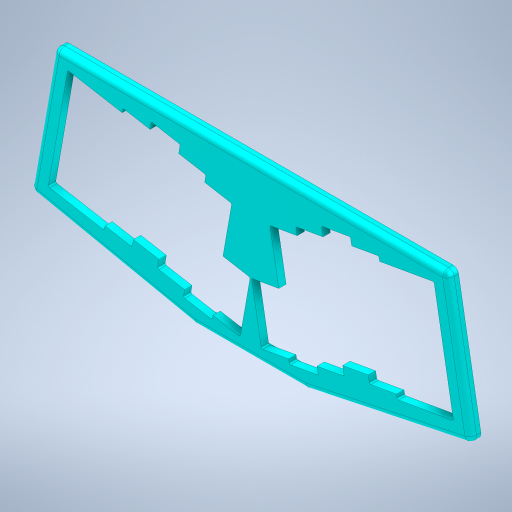
# Autodesk Inventor part: top-case
Saved by Autodesk Inventor 2023 (Build 270158000, 158)
## iProperties
Created: 2022-09-10
Part Number: top-case
Material: Aluminum 6061-AHC
Document SubType Name: Modeling
Designer: hainguyen
Density: 2.7 g/cm^3
Appearance: Aluminum - Dark
Author: hainguyen
Autodesk Inventor part; units mm, degrees
(part 1 of 2)
ref_plane "YZ Plane" through (0, 0, 0) normal (1, 0, 0) x (0, 1, 0)
ref_plane "XZ Plane" through (0, 0, 0) normal (0, 1, 0) x (-1, 0, 0)
ref_plane "XY Plane" through (0, 0, 0) normal (0, 0, 1) x (1, 0, 0)
sketch "Sketch1" plane through (0, 0, 0) normal (0, 0, 1) x (1, 0, 0)
  line L0 (125.9391, 53.8097) -> (-64.6396, 53.8097) construction
  line L1 (191.9239, 53.9833) -> (205.6869, -24.0807) construction
  line L2 (164.2137, -32.7433) -> (204.7021, -24.2544) construction
  line L3 (-64.6396, 53.8097) -> (-78.4038, -24.2539) construction
  line L4 (-78.4038, -24.2539) -> (-37.9155, -32.743) construction
  line L5 (25.7012, -46.0813) -> (100.5969, -46.0813) construction
  line L6 (-72.1915, 62.8097) -> (198.4911, 62.8097)
  line L7 (198.4911, 62.8097) -> (215.0786, -31.2745)
  line L8 (215.0786, -31.2745) -> (101.5302, -55.0813)
  line L9 (101.5302, -55.0813) -> (24.7678, -55.0813)
  line L10 (24.7678, -55.0813) -> (-88.7804, -31.274)
  line L11 (-88.7804, -31.274) -> (-72.1915, 62.8097)
  line L12 (204.7021, -24.2544) -> (190.9391, 53.8097) construction
  point P0 (0, 0)
extrude "Extrusion1" add sketch "Sketch1" along normal blind 7
sketch "Sketch2" plane through (0, 0, 0) normal (0, 0, -1) x (-1, 0, 0)
  arc A0 (47.2919, 31.2612) -> (47.5236, 31.0989) centre (47.4889, 31.2959) ccw construction
  line L0 (65.0532, 34.1898) -> (47.5236, 31.0989) construction
  arc A1 (65.0532, 34.1898) -> (65.2154, 34.4214) centre (65.0185, 34.3867) ccw construction
  line L1 (62.1246, 51.951) -> (65.2154, 34.4214) construction
  arc A2 (62.1246, 51.951) -> (61.8929, 52.1133) centre (61.9276, 51.9163) ccw construction
  line L2 (44.3633, 49.0224) -> (61.8929, 52.1133) construction
  arc A3 (44.3633, 49.0224) -> (44.2011, 48.7907) centre (44.398, 48.8255) ccw construction
  line L3 (47.2919, 31.2612) -> (44.2011, 48.7907) construction
  line L4 (63.1649, 35.6846) -> (48.7867, 33.1494) construction
  line L5 (48.7867, 33.1494) -> (46.2516, 47.5276) construction
  line L6 (46.2516, 47.5276) -> (60.6298, 50.0628) construction
  line L7 (60.6298, 50.0628) -> (63.1649, 35.6846) construction
  arc A4 (28.5806, 27.9618) -> (28.8122, 27.7996) centre (28.7775, 27.9966) ccw construction
  line L8 (46.3418, 30.8904) -> (28.8122, 27.7996) construction
  arc A5 (46.3418, 30.8904) -> (46.5041, 31.1221) centre (46.3071, 31.0874) ccw construction
  line L9 (43.4132, 48.6517) -> (46.5041, 31.1221) construction
  arc A6 (43.4132, 48.6517) -> (43.1816, 48.814) centre (43.2163, 48.617) ccw construction
  line L10 (25.652, 45.7231) -> (43.1816, 48.814) construction
  arc A7 (25.652, 45.7231) -> (25.4897, 45.4914) centre (25.6867, 45.5262) ccw construction
  line L11 (28.5806, 27.9618) -> (25.4897, 45.4914) construction
  line L12 (44.4536, 32.3853) -> (30.0754, 29.8501) construction
  line L13 (30.0754, 29.8501) -> (27.5402, 44.2283) construction
  line L14 (27.5402, 44.2283) -> (41.9184, 46.7635) construction
  line L15 (41.9184, 46.7635) -> (44.4536, 32.3853) construction
  arc A8 (9.3483, 27.6169) -> (9.58, 27.4547) centre (9.5452, 27.6517) ccw construction
  line L16 (27.1096, 30.5455) -> (9.58, 27.4547) construction
  arc A9 (27.1096, 30.5455) -> (27.2718, 30.7772) centre (27.0748, 30.7425) ccw construction
  line L17 (24.1809, 48.3068) -> (27.2718, 30.7772) construction
  arc A10 (24.1809, 48.3068) -> (23.9493, 48.4691) centre (23.984, 48.2721) ccw construction
  line L18 (6.4197, 45.3782) -> (23.9493, 48.4691) construction
  arc A11 (6.4197, 45.3782) -> (6.2574, 45.1465) centre (6.4544, 45.1813) ccw construction
  line L19 (9.3483, 27.6169) -> (6.2574, 45.1465) construction
  line L20 (25.2213, 32.0404) -> (10.8431, 29.5052) construction
  line L21 (10.8431, 29.5052) -> (8.3079, 43.8834) construction
  line L22 (8.3079, 43.8834) -> (22.6861, 46.4186) construction
  line L23 (22.6861, 46.4186) -> (25.2213, 32.0404) construction
  arc A12 (-10.2313, 29.2417) -> (-9.9996, 29.0794) centre (-10.0344, 29.2764) ccw construction
  line L24 (7.53, 32.1703) -> (-9.9996, 29.0794) construction
  arc A13 (7.53, 32.1703) -> (7.6922, 32.402) centre (7.4952, 32.3672) ccw construction
  line L25 (4.6014, 49.9316) -> (7.6922, 32.402) construction
  arc A14 (4.6014, 49.9316) -> (4.3697, 50.0938) centre (4.4044, 49.8968) ccw construction
  line L26 (-13.1599, 47.003) -> (4.3697, 50.0938) construction
  arc A15 (-13.1599, 47.003) -> (-13.3222, 46.7713) centre (-13.1252, 46.806) ccw construction
  line L27 (-10.2313, 29.2417) -> (-13.3222, 46.7713) construction
  line L28 (5.6417, 33.6651) -> (-8.7365, 31.1299) construction
  line L29 (-8.7365, 31.1299) -> (-11.2717, 45.5081) construction
  line L30 (-11.2717, 45.5081) -> (3.1065, 48.0433) construction
  line L31 (3.1065, 48.0433) -> (5.6417, 33.6651) construction
  arc A16 (-27.9008, 20.0335) -> (-27.6691, 19.8713) centre (-27.7038, 20.0682) ccw construction
  line L32 (-10.1395, 22.9621) -> (-27.6691, 19.8713) construction
  arc A17 (-10.1395, 22.9621) -> (-9.9773, 23.1938) centre (-10.1742, 23.1591) ccw construction
  line L33 (-13.0681, 40.7234) -> (-9.9773, 23.1938) construction
  arc A18 (-13.0681, 40.7234) -> (-13.2998, 40.8856) centre (-13.2651, 40.6887) ccw construction
  line L34 (-30.8294, 37.7948) -> (-13.2998, 40.8856) construction
  arc A19 (-30.8294, 37.7948) -> (-30.9916, 37.5631) centre (-30.7947, 37.5978) ccw construction
  line L35 (-27.9008, 20.0335) -> (-30.9916, 37.5631) construction
  line L36 (-12.0277, 24.4569) -> (-26.406, 21.9218) construction
  line L37 (-26.406, 21.9218) -> (-28.9411, 36.3) construction
  line L38 (-28.9411, 36.3) -> (-14.5629, 38.8351) construction
  line L39 (-14.5629, 38.8351) -> (-12.0277, 24.4569) construction
  arc A20 (-45.7439, 11.8102) -> (-45.5122, 11.6479) centre (-45.5469, 11.8449) ccw construction
  line L40 (-27.9826, 14.7388) -> (-45.5122, 11.6479) construction
  arc A21 (-27.9826, 14.7388) -> (-27.8204, 14.9704) centre (-28.0173, 14.9357) ccw construction
  line L41 (-30.9112, 32.5) -> (-27.8204, 14.9704) construction
  arc A22 (-30.9112, 32.5) -> (-31.1429, 32.6623) centre (-31.1082, 32.4653) ccw construction
  line L42 (-48.6725, 29.5714) -> (-31.1429, 32.6623) construction
  arc A23 (-48.6725, 29.5714) -> (-48.8347, 29.3397) centre (-48.6378, 29.3745) ccw construction
  line L43 (-45.7439, 11.8102) -> (-48.8347, 29.3397) construction
  line L44 (-29.8709, 16.2336) -> (-44.2491, 13.6984) construction
  line L45 (-44.2491, 13.6984) -> (-46.7842, 28.0766) construction
  line L46 (-46.7842, 28.0766) -> (-32.406, 30.6118) construction
  line L47 (-32.406, 30.6118) -> (-29.8709, 16.2336) construction
  arc A24 (-55.0778, -44.6518) -> (-54.8461, -44.8141) centre (-54.8809, -44.6171) ccw construction
  line L48 (-37.3165, -41.7232) -> (-54.8461, -44.8141) construction
  arc A25 (-37.3165, -41.7232) -> (-37.1543, -41.4916) centre (-37.3513, -41.5263) ccw construction
  line L49 (-40.2451, -23.962) -> (-37.1543, -41.4916) construction
  arc A26 (-40.2451, -23.962) -> (-40.4768, -23.7997) centre (-40.4421, -23.9967) ccw construction
  line L50 (-58.0064, -26.8906) -> (-40.4768, -23.7997) construction
  arc A27 (-58.0064, -26.8906) -> (-58.1687, -27.1222) centre (-57.9717, -27.0875) ccw construction
  line L51 (-55.0778, -44.6518) -> (-58.1687, -27.1222) construction
  line L52 (-39.2048, -40.2284) -> (-53.583, -42.7636) construction
  line L53 (-53.583, -42.7636) -> (-56.1182, -28.3854) construction
  line L54 (-56.1182, -28.3854) -> (-41.74, -25.8502) construction
  line L55 (-41.74, -25.8502) -> (-39.2048, -40.2284) construction
  arc A28 (-58.3751, -25.9518) -> (-58.1435, -26.1141) centre (-58.1782, -25.9171) ccw construction
  line L56 (-40.6139, -23.0232) -> (-58.1435, -26.1141) construction
  arc A29 (-40.6139, -23.0232) -> (-40.4516, -22.7916) centre (-40.6486, -22.8263) ccw construction
  line L57 (-43.5425, -5.262) -> (-40.4516, -22.7916) construction
  arc A30 (-43.5425, -5.262) -> (-43.7741, -5.0997) centre (-43.7394, -5.2967) ccw construction
  line L58 (-61.3037, -8.1906) -> (-43.7741, -5.0997) construction
  arc A31 (-61.3037, -8.1906) -> (-61.466, -8.4222) centre (-61.269, -8.3875) ccw construction
  line L59 (-58.3751, -25.9518) -> (-61.466, -8.4222) construction
  line L60 (-42.5021, -21.5284) -> (-56.8803, -24.0636) construction
  line L61 (-56.8803, -24.0636) -> (-59.4155, -9.6854) construction
  line L62 (-59.4155, -9.6854) -> (-45.0373, -7.1502) construction
  line L63 (-45.0373, -7.1502) -> (-42.5021, -21.5284) construction
  arc A32 (-35.8459, -44.3239) -> (-35.6143, -44.4861) centre (-35.649, -44.2892) ccw construction
  line L64 (-18.0847, -41.3953) -> (-35.6143, -44.4861) construction
  arc A33 (-18.0847, -41.3953) -> (-17.9224, -41.1636) centre (-18.1194, -41.1983) ccw construction
  line L65 (-21.0133, -23.634) -> (-17.9224, -41.1636) construction
  arc A34 (-21.0133, -23.634) -> (-21.2449, -23.4718) centre (-21.2102, -23.6687) ccw construction
  line L66 (-38.7745, -26.5626) -> (-21.2449, -23.4718) construction
  arc A35 (-38.7745, -26.5626) -> (-38.9368, -26.7943) centre (-38.7398, -26.7596) ccw construction
  line L67 (-35.8459, -44.3239) -> (-38.9368, -26.7943) construction
  line L68 (-19.9729, -39.9005) -> (-34.3511, -42.4356) construction
  line L69 (-34.3511, -42.4356) -> (-36.8863, -28.0574) construction
  line L70 (-36.8863, -28.0574) -> (-22.5081, -25.5223) construction
  line L71 (-22.5081, -25.5223) -> (-19.9729, -39.9005) construction
  arc A36 (-18.0028, -36.1005) -> (-17.7711, -36.2628) centre (-17.8059, -36.0658) ccw construction
  line L72 (-0.2415, -33.1719) -> (-17.7711, -36.2628) construction
  arc A37 (-0.2415, -33.1719) -> (-0.0793, -32.9402) centre (-0.2763, -32.975) ccw construction
  line L73 (-3.1702, -15.4106) -> (-0.0793, -32.9402) construction
  arc A38 (-3.1702, -15.4106) -> (-3.4018, -15.2484) centre (-3.3671, -15.4454) ccw construction
  line L74 (-20.9314, -18.3392) -> (-3.4018, -15.2484) construction
  arc A39 (-20.9314, -18.3392) -> (-21.0937, -18.5709) centre (-20.8967, -18.5362) ccw construction
  line L75 (-18.0028, -36.1005) -> (-21.0937, -18.5709) construction
  line L76 (-2.1298, -31.6771) -> (-16.508, -34.2123) construction
  line L77 (-16.508, -34.2123) -> (-19.0432, -19.8341) construction
  line L78 (-19.0432, -19.8341) -> (-4.665, -17.2989) construction
  line L79 (-4.665, -17.2989) -> (-2.1298, -31.6771) construction
  arc A40 (-0.3334, -26.8924) -> (-0.1017, -27.0546) centre (-0.1364, -26.8576) ccw construction
  line L80 (17.4279, -23.9638) -> (-0.1017, -27.0546) construction
  arc A41 (17.4279, -23.9638) -> (17.5901, -23.7321) centre (17.3932, -23.7668) ccw construction
  line L81 (14.4993, -6.2025) -> (17.5901, -23.7321) construction
  arc A42 (14.4993, -6.2025) -> (14.2676, -6.0403) centre (14.3023, -6.2372) ccw construction
  line L82 (-3.262, -9.1311) -> (14.2676, -6.0403) construction
  arc A43 (-3.262, -9.1311) -> (-3.4242, -9.3628) centre (-3.2273, -9.328) ccw construction
  line L83 (-0.3334, -26.8924) -> (-3.4242, -9.3628) construction
  line L84 (15.5397, -22.4689) -> (1.1615, -25.0041) construction
  line L85 (1.1615, -25.0041) -> (-1.3737, -10.6259) construction
  line L86 (-1.3737, -10.6259) -> (13.0045, -8.0907) construction
  line L87 (13.0045, -8.0907) -> (15.5397, -22.4689) construction
  arc A44 (19.2462, -28.5171) -> (19.4779, -28.6793) centre (19.4432, -28.4824) ccw construction
  line L88 (37.0075, -25.5885) -> (19.4779, -28.6793) construction
  arc A45 (37.0075, -25.5885) -> (37.1697, -25.3568) centre (36.9728, -25.3915) ccw construction
  line L89 (34.0789, -7.8272) -> (37.1697, -25.3568) construction
  arc A46 (34.0789, -7.8272) -> (33.8472, -7.665) centre (33.8819, -7.8619) ccw construction
  line L90 (16.3176, -10.7558) -> (33.8472, -7.665) construction
  arc A47 (16.3176, -10.7558) -> (16.1554, -10.9875) centre (16.3523, -10.9528) ccw construction
  line L91 (19.2462, -28.5171) -> (16.1554, -10.9875) construction
  line L92 (35.1192, -24.0937) -> (20.741, -26.6288) construction
  line L93 (20.741, -26.6288) -> (18.2059, -12.2506) construction
  line L94 (18.2059, -12.2506) -> (32.5841, -9.7155) construction
  line L95 (32.5841, -9.7155) -> (35.1192, -24.0937) construction
  arc A48 (38.4785, -28.1722) -> (38.7102, -28.3344) centre (38.6755, -28.1375) ccw construction
  line L96 (56.2398, -25.2436) -> (38.7102, -28.3344) construction
  arc A49 (56.2398, -25.2436) -> (56.402, -25.0119) centre (56.2051, -25.0466) ccw construction
  line L97 (53.3112, -7.4823) -> (56.402, -25.0119) construction
  arc A50 (53.3112, -7.4823) -> (53.0795, -7.3201) centre (53.1142, -7.517) ccw construction
  line L98 (35.5499, -10.4109) -> (53.0795, -7.3201) construction
  arc A51 (35.5499, -10.4109) -> (35.3877, -10.6426) centre (35.5846, -10.6079) ccw construction
  line L99 (38.4785, -28.1722) -> (35.3877, -10.6426) construction
  line L100 (54.3515, -23.7488) -> (39.9733, -26.284) construction
  line L101 (39.9733, -26.284) -> (37.4382, -11.9057) construction
  line L102 (37.4382, -11.9057) -> (51.8164, -9.3706) construction
  line L103 (51.8164, -9.3706) -> (54.3515, -23.7488) construction
  arc A52 (57.1899, -24.8729) -> (57.4215, -25.0351) centre (57.3868, -24.8382) ccw construction
  line L104 (74.9511, -21.9443) -> (57.4215, -25.0351) construction
  arc A53 (74.9511, -21.9443) -> (75.1134, -21.7126) centre (74.9164, -21.7473) ccw construction
  line L105 (72.0225, -4.183) -> (75.1134, -21.7126) construction
  arc A54 (72.0225, -4.183) -> (71.7908, -4.0208) centre (71.8256, -4.2177) ccw construction
  line L106 (54.2612, -7.1116) -> (71.7908, -4.0208) construction
  arc A55 (54.2612, -7.1116) -> (54.099, -7.3433) centre (54.296, -7.3086) ccw construction
  line L107 (57.1899, -24.8729) -> (54.099, -7.3433) construction
  line L108 (73.0629, -20.4495) -> (58.6847, -22.9846) construction
  line L109 (58.6847, -22.9846) -> (56.1495, -8.6064) construction
  line L110 (56.1495, -8.6064) -> (70.5277, -6.0713) construction
  line L111 (70.5277, -6.0713) -> (73.0629, -20.4495) construction
  arc A56 (-88.9737, -41.5091) -> (-88.8115, -41.7408) centre (-88.7767, -41.5438) ccw construction
  line L112 (-71.2818, -44.8313) -> (-88.8115, -41.7408) construction
  arc A57 (-71.2818, -44.8313) -> (-71.0501, -44.6691) centre (-71.2471, -44.6344) ccw construction
  line L113 (-67.9596, -27.1394) -> (-71.0501, -44.6691) construction
  arc A58 (-67.9596, -27.1394) -> (-68.1218, -26.9078) centre (-68.1565, -27.1047) ccw construction
  line L114 (-85.6515, -23.8172) -> (-68.1218, -26.9078) construction
  arc A59 (-85.6515, -23.8172) -> (-85.8832, -23.9794) centre (-85.6862, -24.0142) ccw construction
  line L115 (-88.9737, -41.5091) -> (-85.8832, -23.9794) construction
  line L116 (-72.545, -42.7809) -> (-86.9232, -40.2459) construction
  line L117 (-86.9232, -40.2459) -> (-84.3883, -25.8677) construction
  line L118 (-84.3883, -25.8677) -> (-70.01, -28.4026) construction
  line L119 (-70.01, -28.4026) -> (-72.545, -42.7809) construction
  arc A60 (-108.2002, -41.175) -> (-108.038, -41.4067) centre (-108.0033, -41.2098) ccw construction
  line L120 (-90.5084, -44.4973) -> (-108.038, -41.4067) construction
  arc A61 (-90.5084, -44.4973) -> (-90.2767, -44.335) centre (-90.4736, -44.3003) ccw construction
  line L121 (-87.1861, -26.8054) -> (-90.2767, -44.335) construction
  arc A62 (-87.1861, -26.8054) -> (-87.3484, -26.5737) centre (-87.3831, -26.7707) ccw construction
  line L122 (-104.878, -23.4831) -> (-87.3484, -26.5737) construction
  arc A63 (-104.878, -23.4831) -> (-105.1097, -23.6454) centre (-104.9127, -23.6801) ccw construction
  line L123 (-108.2002, -41.175) -> (-105.1097, -23.6454) construction
  line L124 (-91.7715, -42.4468) -> (-106.1498, -39.9119) construction
  line L125 (-106.1498, -39.9119) -> (-103.6148, -25.5336) construction
  line L126 (-103.6148, -25.5336) -> (-89.2366, -28.0686) construction
  line L127 (-89.2366, -28.0686) -> (-91.7715, -42.4468) construction
  arc A64 (-126.0433, -32.9517) -> (-125.8811, -33.1834) centre (-125.8464, -32.9864) ccw construction
  line L128 (-108.3515, -36.2739) -> (-125.8811, -33.1834) construction
  arc A65 (-108.3515, -36.2739) -> (-108.1198, -36.1117) centre (-108.3167, -36.077) ccw construction
  line L129 (-105.0292, -18.582) -> (-108.1198, -36.1117) construction
  arc A66 (-105.0292, -18.582) -> (-105.1915, -18.3503) centre (-105.2262, -18.5473) ccw construction
  line L130 (-122.7211, -15.2598) -> (-105.1915, -18.3503) construction
  arc A67 (-122.7211, -15.2598) -> (-122.9528, -15.422) centre (-122.7558, -15.4568) ccw construction
  line L131 (-126.0433, -32.9517) -> (-122.9528, -15.422) construction
  line L132 (-109.6146, -34.2235) -> (-123.9929, -31.6885) construction
  line L133 (-123.9929, -31.6885) -> (-121.4579, -17.3103) construction
  line L134 (-121.4579, -17.3103) -> (-107.0797, -19.8452) construction
  line L135 (-107.0797, -19.8452) -> (-109.6146, -34.2235) construction
  arc A68 (-143.7128, -23.7435) -> (-143.5506, -23.9752) centre (-143.5158, -23.7782) ccw construction
  line L136 (-126.0209, -27.0658) -> (-143.5506, -23.9752) construction
  arc A69 (-126.0209, -27.0658) -> (-125.7892, -26.9035) centre (-125.9862, -26.8688) ccw construction
  line L137 (-122.6987, -9.3739) -> (-125.7892, -26.9035) construction
  arc A70 (-122.6987, -9.3739) -> (-122.8609, -9.1422) centre (-122.8956, -9.3391) ccw construction
  line L138 (-140.3906, -6.0516) -> (-122.8609, -9.1422) construction
  arc A71 (-140.3906, -6.0516) -> (-140.6223, -6.2139) centre (-140.4253, -6.2486) ccw construction
  line L139 (-143.7128, -23.7435) -> (-140.6223, -6.2139) construction
  line L140 (-127.2841, -25.0153) -> (-141.6623, -22.4803) construction
  line L141 (-141.6623, -22.4803) -> (-139.1274, -8.1021) construction
  line L142 (-139.1274, -8.1021) -> (-124.7491, -10.637) construction
  line L143 (-124.7491, -10.637) -> (-127.2841, -25.0153) construction
  arc A72 (-163.2924, -25.3682) -> (-163.1302, -25.5999) centre (-163.0954, -25.403) ccw construction
  line L144 (-145.6005, -28.6905) -> (-163.1302, -25.5999) construction
  arc A73 (-145.6005, -28.6905) -> (-145.3688, -28.5282) centre (-145.5658, -28.4935) ccw construction
  line L145 (-142.2783, -10.9986) -> (-145.3688, -28.5282) construction
  arc A74 (-142.2783, -10.9986) -> (-142.4405, -10.7669) centre (-142.4752, -10.9639) ccw construction
  line L146 (-159.9702, -7.6764) -> (-142.4405, -10.7669) construction
  arc A75 (-159.9702, -7.6764) -> (-160.2018, -7.8386) centre (-160.0049, -7.8733) ccw construction
  line L147 (-163.2924, -25.3682) -> (-160.2018, -7.8386) construction
  line L148 (-146.8637, -26.64) -> (-161.2419, -24.1051) construction
  line L149 (-161.2419, -24.1051) -> (-158.707, -9.7268) construction
  line L150 (-158.707, -9.7268) -> (-144.3287, -12.2618) construction
  line L151 (-144.3287, -12.2618) -> (-146.8637, -26.64) construction
  arc A76 (-182.5247, -25.0233) -> (-182.3624, -25.255) centre (-182.3277, -25.0581) ccw construction
  line L152 (-164.8328, -28.3456) -> (-182.3624, -25.255) construction
  arc A77 (-164.8328, -28.3456) -> (-164.6011, -28.1833) centre (-164.7981, -28.1486) ccw construction
  line L153 (-161.5106, -10.6537) -> (-164.6011, -28.1833) construction
  arc A78 (-161.5106, -10.6537) -> (-161.6728, -10.422) centre (-161.7075, -10.619) ccw construction
  line L154 (-179.2024, -7.3315) -> (-161.6728, -10.422) construction
  arc A79 (-179.2024, -7.3315) -> (-179.4341, -7.4937) centre (-179.2372, -7.5284) ccw construction
  line L155 (-182.5247, -25.0233) -> (-179.4341, -7.4937) construction
  line L156 (-166.096, -26.2951) -> (-180.4742, -23.7602) construction
  line L157 (-180.4742, -23.7602) -> (-177.9393, -9.3819) construction
  line L158 (-177.9393, -9.3819) -> (-163.561, -11.9169) construction
  line L159 (-163.561, -11.9169) -> (-166.096, -26.2951) construction
  arc A80 (-201.236, -21.724) -> (-201.0738, -21.9557) centre (-201.0391, -21.7588) ccw construction
  line L160 (-183.5442, -25.0463) -> (-201.0738, -21.9557) construction
  arc A81 (-183.5442, -25.0463) -> (-183.3125, -24.884) centre (-183.5094, -24.8493) ccw construction
  line L161 (-180.2219, -7.3544) -> (-183.3125, -24.884) construction
  arc A82 (-180.2219, -7.3544) -> (-180.3842, -7.1227) centre (-180.4189, -7.3197) ccw construction
  line L162 (-197.9138, -4.0321) -> (-180.3842, -7.1227) construction
  arc A83 (-197.9138, -4.0321) -> (-198.1455, -4.1944) centre (-197.9485, -4.2291) ccw construction
  line L163 (-201.236, -21.724) -> (-198.1455, -4.1944) construction
  line L164 (-184.8073, -22.9958) -> (-199.1856, -20.4609) construction
  line L165 (-199.1856, -20.4609) -> (-196.6506, -6.0826) construction
  line L166 (-196.6506, -6.0826) -> (-182.2724, -8.6176) construction
  line L167 (-182.2724, -8.6176) -> (-184.8073, -22.9958) construction
  arc A84 (-191.3381, 34.41) -> (-191.1759, 34.1783) centre (-191.1411, 34.3753) ccw construction
  line L168 (-173.6462, 31.0878) -> (-191.1759, 34.1783) construction
  arc A85 (-173.6462, 31.0878) -> (-173.4145, 31.25) centre (-173.6115, 31.2847) ccw construction
  line L169 (-170.324, 48.7797) -> (-173.4145, 31.25) construction
  arc A86 (-170.324, 48.7797) -> (-170.4862, 49.0113) centre (-170.5209, 48.8144) ccw construction
  line L170 (-188.0158, 52.1019) -> (-170.4862, 49.0113) construction
  arc A87 (-188.0158, 52.1019) -> (-188.2475, 51.9397) centre (-188.0506, 51.9049) ccw construction
  line L171 (-191.3381, 34.41) -> (-188.2475, 51.9397) construction
  line L172 (-174.9094, 33.1382) -> (-189.2876, 35.6732) construction
  line L173 (-189.2876, 35.6732) -> (-186.7527, 50.0514) construction
  line L174 (-186.7527, 50.0514) -> (-172.3744, 47.5165) construction
  line L175 (-172.3744, 47.5165) -> (-174.9094, 33.1382) construction
  arc A88 (-172.6267, 31.1107) -> (-172.4645, 30.879) centre (-172.4298, 31.076) ccw construction
  line L176 (-154.9349, 27.7885) -> (-172.4645, 30.879) construction
  arc A89 (-154.9349, 27.7885) -> (-154.7032, 27.9507) centre (-154.9001, 27.9854) ccw construction
  line L177 (-151.6126, 45.4803) -> (-154.7032, 27.9507) construction
  arc A90 (-151.6126, 45.4803) -> (-151.7749, 45.712) centre (-151.8096, 45.5151) ccw construction
  line L178 (-169.3045, 48.8026) -> (-151.7749, 45.712) construction
  arc A91 (-169.3045, 48.8026) -> (-169.5362, 48.6403) centre (-169.3392, 48.6056) ccw construction
  line L179 (-172.6267, 31.1107) -> (-169.5362, 48.6403) construction
  line L180 (-156.198, 29.8389) -> (-170.5763, 32.3739) construction
  line L181 (-170.5763, 32.3739) -> (-168.0413, 46.7521) construction
  line L182 (-168.0413, 46.7521) -> (-153.6631, 44.2172) construction
  line L183 (-153.6631, 44.2172) -> (-156.198, 29.8389) construction
  arc A92 (-153.3944, 30.7658) -> (-153.2322, 30.5341) centre (-153.1975, 30.7311) ccw construction
  line L184 (-135.7026, 27.4436) -> (-153.2322, 30.5341) construction
  arc A93 (-135.7026, 27.4436) -> (-135.4709, 27.6058) centre (-135.6678, 27.6405) ccw construction
  line L185 (-132.3803, 45.1354) -> (-135.4709, 27.6058) construction
  arc A94 (-132.3803, 45.1354) -> (-132.5426, 45.3671) centre (-132.5773, 45.1702) ccw construction
  line L186 (-150.0722, 48.4577) -> (-132.5426, 45.3671) construction
  arc A95 (-150.0722, 48.4577) -> (-150.3039, 48.2954) centre (-150.1069, 48.2607) ccw construction
  line L187 (-153.3944, 30.7658) -> (-150.3039, 48.2954) construction
  line L188 (-136.9657, 29.494) -> (-151.344, 32.029) construction
  line L189 (-151.344, 32.029) -> (-148.809, 46.4072) construction
  line L190 (-148.809, 46.4072) -> (-134.4308, 43.8723) construction
  line L191 (-134.4308, 43.8723) -> (-136.9657, 29.494) construction
  arc A96 (-133.8149, 32.3905) -> (-133.6526, 32.1588) centre (-133.6179, 32.3558) ccw construction
  line L192 (-116.123, 29.0683) -> (-133.6526, 32.1588) construction
  arc A97 (-116.123, 29.0683) -> (-115.8913, 29.2305) centre (-116.0883, 29.2652) ccw construction
  line L193 (-112.8007, 46.7602) -> (-115.8913, 29.2305) construction
  arc A98 (-112.8007, 46.7602) -> (-112.963, 46.9919) centre (-112.9977, 46.7949) ccw construction
  line L194 (-130.4926, 50.0824) -> (-112.963, 46.9919) construction
  arc A99 (-130.4926, 50.0824) -> (-130.7243, 49.9202) centre (-130.5273, 49.8854) ccw construction
  line L195 (-133.8149, 32.3905) -> (-130.7243, 49.9202) construction
  line L196 (-117.3861, 31.1188) -> (-131.7644, 33.6537) construction
  line L197 (-131.7644, 33.6537) -> (-129.2295, 48.0319) construction
  line L198 (-129.2295, 48.0319) -> (-114.8512, 45.497) construction
  line L199 (-114.8512, 45.497) -> (-117.3861, 31.1188) construction
  arc A100 (-116.1454, 23.1824) -> (-115.9832, 22.9507) centre (-115.9484, 23.1476) ccw construction
  line L200 (-98.4535, 19.8601) -> (-115.9832, 22.9507) construction
  arc A101 (-98.4535, 19.8601) -> (-98.2218, 20.0224) centre (-98.4188, 20.0571) ccw construction
  line L201 (-95.1313, 37.552) -> (-98.2218, 20.0224) construction
  arc A102 (-95.1313, 37.552) -> (-95.2935, 37.7837) centre (-95.3282, 37.5867) ccw construction
  line L202 (-112.8232, 40.8742) -> (-95.2935, 37.7837) construction
  arc A103 (-112.8232, 40.8742) -> (-113.0549, 40.712) centre (-112.8579, 40.6773) ccw construction
  line L203 (-116.1454, 23.1824) -> (-113.0549, 40.712) construction
  line L204 (-99.7167, 21.9106) -> (-114.0949, 24.4455) construction
  line L205 (-114.0949, 24.4455) -> (-111.56, 38.8238) construction
  line L206 (-111.56, 38.8238) -> (-97.1817, 36.2888) construction
  line L207 (-97.1817, 36.2888) -> (-99.7167, 21.9106) construction
  arc A104 (-98.3023, 14.959) -> (-98.1401, 14.7273) centre (-98.1053, 14.9243) ccw construction
  line L208 (-80.6104, 11.6368) -> (-98.1401, 14.7273) construction
  arc A105 (-80.6104, 11.6368) -> (-80.3787, 11.799) centre (-80.5757, 11.8337) ccw construction
  line L209 (-77.2882, 29.3287) -> (-80.3787, 11.799) construction
  arc A106 (-77.2882, 29.3287) -> (-77.4504, 29.5603) centre (-77.4851, 29.3634) ccw construction
  line L210 (-94.9801, 32.6509) -> (-77.4504, 29.5603) construction
  arc A107 (-94.9801, 32.6509) -> (-95.2117, 32.4887) centre (-95.0148, 32.4539) ccw construction
  line L211 (-98.3023, 14.959) -> (-95.2117, 32.4887) construction
  line L212 (-81.8736, 13.6872) -> (-96.2518, 16.2222) construction
  line L213 (-96.2518, 16.2222) -> (-93.7169, 30.6004) construction
  line L214 (-93.7169, 30.6004) -> (-79.3386, 28.0655) construction
  line L215 (-79.3386, 28.0655) -> (-81.8736, 13.6872) construction
  line L216 (62.9014, 53.3064) -> (25.4783, 46.7079)
  line L217 (25.4783, 46.7079) -> (24.9574, 49.6622)
  line L218 (24.9574, 49.6622) -> (6.246, 46.363)
  line L219 (6.246, 46.363) -> (5.3778, 51.287)
  line L220 (5.3778, 51.287) -> (-14.5153, 47.7794)
  line L221 (-14.5153, 47.7794) -> (-13.4735, 41.8704)
  line L222 (-13.4735, 41.8704) -> (-32.1848, 38.5712)
  line L223 (-32.1848, 38.5712) -> (-31.3166, 33.6471)
  line L224 (-31.3166, 33.6471) -> (-50.0279, 30.3479)
  line L225 (-50.0279, 30.3479) -> (-43.9513, -4.1155)
  line L226 (-43.9513, -4.1155) -> (-62.6592, -7.4141)
  line L227 (62.9014, 53.3064) -> (76.3066, -22.7207)
  line L228 (76.3066, -22.7207) -> (37.702, -29.5275)
  line L229 (37.702, -29.5275) -> (37.1812, -26.5733)
  line L230 (37.1812, -26.5733) -> (18.5275, -29.8623)
  line L231 (18.5275, -29.8623) -> (17.6593, -24.9384)
  line L232 (17.6593, -24.9384) -> (0.072, -28.0394)
  line L233 (0.072, -28.0394) -> (1.1139, -33.9484)
  line L234 (1.1139, -33.9484) -> (-17.5975, -37.2476)
  line L235 (-17.5975, -37.2476) -> (-16.7292, -42.1717)
  line L236 (-16.7292, -42.1717) -> (-36.6224, -45.6793)
  line L237 (-37.1462, -42.7086) -> (-55.8544, -46.0073)
  line L238 (-36.6224, -45.6793) -> (-37.1462, -42.7086)
  line L239 (-62.6592, -7.4141) -> (-55.8544, -46.0073)
  line L240 (-63.1489, -68.009) -> (-63.1501, 79.9495) construction
  arc A108 (-173.8231, 31.0971) -> (-173.5914, 31.2594) centre (-173.7883, 31.2941) ccw construction
  line L241 (-191.3527, 34.1877) -> (-173.8231, 31.0971) construction
  arc A109 (-191.515, 34.4194) -> (-191.3527, 34.1877) centre (-191.318, 34.3846) ccw construction
  line L242 (-188.4244, 51.949) -> (-191.515, 34.4194) construction
  arc A110 (-188.1927, 52.1113) -> (-188.4244, 51.949) centre (-188.2274, 51.9143) ccw construction
  line L243 (-170.6631, 49.0207) -> (-188.1927, 52.1113) construction
  arc A111 (-170.5008, 48.789) -> (-170.6631, 49.0207) centre (-170.6978, 48.8237) ccw construction
  line L244 (-173.5914, 31.2594) -> (-170.5008, 48.789) construction
  line L245 (-189.4645, 35.6825) -> (-175.0862, 33.1476) construction
  line L246 (-175.0862, 33.1476) -> (-172.5513, 47.5258) construction
  line L247 (-172.5513, 47.5258) -> (-186.9295, 50.0608) construction
  line L248 (-186.9295, 50.0608) -> (-189.4645, 35.6825) construction
  arc A112 (-155.1117, 27.7981) -> (-154.88, 27.9604) centre (-155.0769, 27.9951) ccw construction
  line L249 (-172.6413, 30.8887) -> (-155.1117, 27.7981) construction
  arc A113 (-172.8036, 31.1204) -> (-172.6413, 30.8887) centre (-172.6066, 31.0856) ccw construction
  line L250 (-169.713, 48.65) -> (-172.8036, 31.1204) construction
  arc A114 (-169.4813, 48.8122) -> (-169.713, 48.65) centre (-169.516, 48.6153) ccw construction
  line L251 (-151.9517, 45.7217) -> (-169.4813, 48.8122) construction
  arc A115 (-151.7894, 45.49) -> (-151.9517, 45.7217) centre (-151.9864, 45.5247) ccw construction
  line L252 (-154.88, 27.9604) -> (-151.7894, 45.49) construction
  line L253 (-170.7531, 32.3835) -> (-156.3748, 29.8486) construction
  line L254 (-156.3748, 29.8486) -> (-153.8399, 44.2268) construction
  line L255 (-153.8399, 44.2268) -> (-168.2181, 46.7618) construction
  line L256 (-168.2181, 46.7618) -> (-170.7531, 32.3835) construction
  arc A116 (-135.8794, 27.4535) -> (-135.6477, 27.6158) centre (-135.8447, 27.6505) ccw construction
  line L257 (-153.409, 30.5441) -> (-135.8794, 27.4535) construction
  arc A117 (-153.5713, 30.7758) -> (-153.409, 30.5441) centre (-153.3743, 30.7411) ccw construction
  line L258 (-150.4807, 48.3054) -> (-153.5713, 30.7758) construction
  arc A118 (-150.249, 48.4677) -> (-150.4807, 48.3054) centre (-150.2837, 48.2707) ccw construction
  line L259 (-132.7194, 45.3771) -> (-150.249, 48.4677) construction
  arc A119 (-132.5571, 45.1454) -> (-132.7194, 45.3771) centre (-132.7541, 45.1801) ccw construction
  line L260 (-135.6477, 27.6158) -> (-132.5571, 45.1454) construction
  line L261 (-151.5208, 32.0389) -> (-137.1425, 29.504) construction
  line L262 (-137.1425, 29.504) -> (-134.6076, 43.8823) construction
  line L263 (-134.6076, 43.8823) -> (-148.9858, 46.4172) construction
  line L264 (-148.9858, 46.4172) -> (-151.5208, 32.0389) construction
  arc A120 (-116.2998, 29.0786) -> (-116.0681, 29.2408) centre (-116.2651, 29.2755) ccw construction
  line L265 (-133.8295, 32.1691) -> (-116.2998, 29.0786) construction
  arc A121 (-133.9917, 32.4008) -> (-133.8295, 32.1691) centre (-133.7947, 32.3661) ccw construction
  line L266 (-130.9011, 49.9305) -> (-133.9917, 32.4008) construction
  arc A122 (-130.6695, 50.0927) -> (-130.9011, 49.9305) centre (-130.7042, 49.8957) ccw construction
  line L267 (-113.1398, 47.0021) -> (-130.6695, 50.0927) construction
  arc A123 (-112.9776, 46.7705) -> (-113.1398, 47.0021) centre (-113.1745, 46.8052) ccw construction
  line L268 (-116.0681, 29.2408) -> (-112.9776, 46.7705) construction
  line L269 (-131.9412, 33.664) -> (-117.563, 31.129) construction
  line L270 (-117.563, 31.129) -> (-115.028, 45.5073) construction
  line L271 (-115.028, 45.5073) -> (-129.4063, 48.0422) construction
  line L272 (-129.4063, 48.0422) -> (-131.9412, 33.664) construction
  arc A124 (-98.6302, 19.8707) -> (-98.3985, 20.0329) centre (-98.5955, 20.0677) ccw construction
  line L273 (-116.1599, 22.9613) -> (-98.6302, 19.8707) construction
  arc A125 (-116.3221, 23.1929) -> (-116.1599, 22.9613) centre (-116.1251, 23.1582) ccw construction
  line L274 (-113.2315, 40.7226) -> (-116.3221, 23.1929) construction
  arc A126 (-112.9999, 40.8848) -> (-113.2315, 40.7226) centre (-113.0346, 40.6879) ccw construction
  line L275 (-95.4702, 37.7943) -> (-112.9999, 40.8848) construction
  arc A127 (-95.308, 37.5626) -> (-95.4702, 37.7943) centre (-95.5049, 37.5973) ccw construction
  line L276 (-98.3985, 20.0329) -> (-95.308, 37.5626) construction
  line L277 (-114.2716, 24.4561) -> (-99.8934, 21.9212) construction
  line L278 (-99.8934, 21.9212) -> (-97.3584, 36.2994) construction
  line L279 (-97.3584, 36.2994) -> (-111.7367, 38.8344) construction
  line L280 (-111.7367, 38.8344) -> (-114.2716, 24.4561) construction
  arc A128 (-80.787, 11.6476) -> (-80.5553, 11.8099) centre (-80.7522, 11.8446) ccw construction
  line L281 (-98.3166, 14.7382) -> (-80.787, 11.6476) construction
  arc A129 (-98.4789, 14.9699) -> (-98.3166, 14.7382) centre (-98.2819, 14.9351) ccw construction
  line L282 (-95.3883, 32.4995) -> (-98.4789, 14.9699) construction
  arc A130 (-95.1566, 32.6618) -> (-95.3883, 32.4995) centre (-95.1913, 32.4648) ccw construction
  line L283 (-77.627, 29.5712) -> (-95.1566, 32.6618) construction
  arc A131 (-77.4647, 29.3395) -> (-77.627, 29.5712) centre (-77.6617, 29.3742) ccw construction
  line L284 (-80.5553, 11.8099) -> (-77.4647, 29.3395) construction
  line L285 (-96.4284, 16.233) -> (-82.0501, 13.6981) construction
  line L286 (-82.0501, 13.6981) -> (-79.5152, 28.0763) construction
  line L287 (-79.5152, 28.0763) -> (-93.8934, 30.6113) construction
  line L288 (-93.8934, 30.6113) -> (-96.4284, 16.233) construction
  arc A132 (-71.4521, -44.8142) -> (-71.2204, -44.652) centre (-71.4174, -44.6172) ccw construction
  line L289 (-88.9818, -41.7237) -> (-71.4521, -44.8142) construction
  arc A133 (-89.144, -41.492) -> (-88.9818, -41.7237) centre (-88.947, -41.5267) ccw construction
  line L290 (-86.0534, -23.9623) -> (-89.144, -41.492) construction
  arc A134 (-85.8218, -23.8001) -> (-86.0534, -23.9623) centre (-85.8565, -23.997) ccw construction
  line L291 (-68.2921, -26.8906) -> (-85.8218, -23.8001) construction
  arc A135 (-68.1299, -27.1223) -> (-68.2921, -26.8906) centre (-68.3268, -27.0876) ccw construction
  line L292 (-71.2204, -44.652) -> (-68.1299, -27.1223) construction
  line L293 (-87.0935, -40.2288) -> (-72.7153, -42.7637) construction
  line L294 (-72.7153, -42.7637) -> (-70.1803, -28.3855) construction
  line L295 (-70.1803, -28.3855) -> (-84.5586, -25.8506) construction
  line L296 (-84.5586, -25.8506) -> (-87.0935, -40.2288) construction
  arc A136 (-68.1551, -26.1142) -> (-67.9234, -25.9519) centre (-68.1204, -25.9172) ccw construction
  line L297 (-85.6848, -23.0236) -> (-68.1551, -26.1142) construction
  arc A137 (-85.847, -22.7919) -> (-85.6848, -23.0236) centre (-85.65, -22.8266) ccw construction
  line L298 (-82.7564, -5.2623) -> (-85.847, -22.7919) construction
  arc A138 (-82.5248, -5.1) -> (-82.7564, -5.2623) centre (-82.5595, -5.297) ccw construction
  line L299 (-64.9951, -8.1906) -> (-82.5248, -5.1) construction
  arc A139 (-64.8329, -8.4223) -> (-64.9951, -8.1906) centre (-65.0298, -8.3875) ccw construction
  line L300 (-67.9234, -25.9519) -> (-64.8329, -8.4223) construction
  line L301 (-83.7965, -21.5287) -> (-69.4183, -24.0637) construction
  line L302 (-69.4183, -24.0637) -> (-66.8833, -9.6854) construction
  line L303 (-66.8833, -9.6854) -> (-81.2616, -7.1505) construction
  line L304 (-81.2616, -7.1505) -> (-83.7965, -21.5287) construction
  arc A140 (-90.684, -44.4866) -> (-90.4523, -44.3243) centre (-90.6493, -44.2896) ccw construction
  line L305 (-108.2137, -41.396) -> (-90.684, -44.4866) construction
  arc A141 (-108.3759, -41.1643) -> (-108.2137, -41.396) centre (-108.1789, -41.1991) ccw construction
  line L306 (-105.2853, -23.6347) -> (-108.3759, -41.1643) construction
  arc A142 (-105.0537, -23.4724) -> (-105.2853, -23.6347) centre (-105.0884, -23.6694) ccw construction
  line L307 (-87.524, -26.563) -> (-105.0537, -23.4724) construction
  arc A143 (-87.3618, -26.7947) -> (-87.524, -26.563) centre (-87.5587, -26.76) ccw construction
  line L308 (-90.4523, -44.3243) -> (-87.3618, -26.7947) construction
  line L309 (-106.3254, -39.9012) -> (-91.9472, -42.4361) construction
  line L310 (-91.9472, -42.4361) -> (-89.4122, -28.0579) construction
  line L311 (-89.4122, -28.0579) -> (-103.7905, -25.5229) construction
  line L312 (-103.7905, -25.5229) -> (-106.3254, -39.9012) construction
  arc A144 (-108.5272, -36.2635) -> (-108.2956, -36.1013) centre (-108.4925, -36.0665) ccw construction
  line L313 (-126.0569, -33.1729) -> (-108.5272, -36.2635) construction
  arc A145 (-126.2191, -32.9413) -> (-126.0569, -33.1729) centre (-126.0222, -32.976) ccw construction
  line L314 (-123.1286, -15.4116) -> (-126.2191, -32.9413) construction
  arc A146 (-122.8969, -15.2494) -> (-123.1286, -15.4116) centre (-122.9316, -15.4463) ccw construction
  line L315 (-105.3672, -18.3399) -> (-122.8969, -15.2494) construction
  arc A147 (-105.205, -18.5716) -> (-105.3672, -18.3399) centre (-105.402, -18.5369) ccw construction
  line L316 (-108.2956, -36.1013) -> (-105.205, -18.5716) construction
  line L317 (-124.1687, -31.6781) -> (-109.7904, -34.213) construction
  line L318 (-109.7904, -34.213) -> (-107.2555, -19.8348) construction
  line L319 (-107.2555, -19.8348) -> (-121.6337, -17.2998) construction
  line L320 (-121.6337, -17.2998) -> (-124.1687, -31.6781) construction
  arc A148 (-126.1969, -27.0556) -> (-125.9652, -26.8934) centre (-126.1621, -26.8587) ccw construction
  line L321 (-143.7265, -23.9651) -> (-126.1969, -27.0556) construction
  arc A149 (-143.8887, -23.7334) -> (-143.7265, -23.9651) centre (-143.6918, -23.7681) ccw construction
  line L322 (-140.7982, -6.2037) -> (-143.8887, -23.7334) construction
  arc A150 (-140.5665, -6.0415) -> (-140.7982, -6.2037) centre (-140.6012, -6.2385) ccw construction
  line L323 (-123.0369, -9.1321) -> (-140.5665, -6.0415) construction
  arc A151 (-122.8746, -9.3637) -> (-123.0369, -9.1321) centre (-123.0716, -9.329) ccw construction
  line L324 (-125.9652, -26.8934) -> (-122.8746, -9.3637) construction
  line L325 (-141.8383, -22.4702) -> (-127.46, -25.0052) construction
  line L326 (-127.46, -25.0052) -> (-124.9251, -10.6269) construction
  line L327 (-124.9251, -10.6269) -> (-139.3033, -8.092) construction
  line L328 (-139.3033, -8.092) -> (-141.8383, -22.4702) construction
  arc A152 (-145.7764, -28.6807) -> (-145.5447, -28.5184) centre (-145.7417, -28.4837) ccw construction
  line L329 (-163.3061, -25.5901) -> (-145.7764, -28.6807) construction
  arc A153 (-163.4683, -25.3584) -> (-163.3061, -25.5901) centre (-163.2713, -25.3931) ccw construction
  line L330 (-160.3777, -7.8288) -> (-163.4683, -25.3584) construction
  arc A154 (-160.1461, -7.6665) -> (-160.3777, -7.8288) centre (-160.1808, -7.8635) ccw construction
  line L331 (-142.6164, -10.7571) -> (-160.1461, -7.6665) construction
  arc A155 (-142.4542, -10.9888) -> (-142.6164, -10.7571) centre (-142.6511, -10.9541) ccw construction
  line L332 (-145.5447, -28.5184) -> (-142.4542, -10.9888) construction
  line L333 (-161.4178, -24.0953) -> (-147.0396, -26.6302) construction
  line L334 (-147.0396, -26.6302) -> (-144.5046, -12.252) construction
  line L335 (-144.5046, -12.252) -> (-158.8829, -9.717) construction
  line L336 (-158.8829, -9.717) -> (-161.4178, -24.0953) construction
  arc A156 (-165.0087, -28.3361) -> (-164.777, -28.1738) centre (-164.974, -28.1391) ccw construction
  line L337 (-182.5384, -25.2455) -> (-165.0087, -28.3361) construction
  arc A157 (-182.7006, -25.0138) -> (-182.5384, -25.2455) centre (-182.5036, -25.0486) ccw construction
  line L338 (-179.61, -7.4842) -> (-182.7006, -25.0138) construction
  arc A158 (-179.3784, -7.322) -> (-179.61, -7.4842) centre (-179.4131, -7.5189) ccw construction
  line L339 (-161.8487, -10.4125) -> (-179.3784, -7.322) construction
  arc A159 (-161.6865, -10.6442) -> (-161.8487, -10.4125) centre (-161.8834, -10.6095) ccw construction
  line L340 (-164.777, -28.1738) -> (-161.6865, -10.6442) construction
  line L341 (-180.6501, -23.7507) -> (-166.2719, -26.2856) construction
  line L342 (-166.2719, -26.2856) -> (-163.7369, -11.9074) construction
  line L343 (-163.7369, -11.9074) -> (-178.1152, -9.3724) construction
  line L344 (-178.1152, -9.3724) -> (-180.6501, -23.7507) construction
  arc A160 (-183.7201, -25.0371) -> (-183.4884, -24.8748) centre (-183.6854, -24.8401) ccw construction
  line L345 (-201.2498, -21.9465) -> (-183.7201, -25.0371) construction
  arc A161 (-201.412, -21.7148) -> (-201.2498, -21.9465) centre (-201.215, -21.7496) ccw construction
  line L346 (-198.3214, -4.1852) -> (-201.412, -21.7148) construction
  arc A162 (-198.0898, -4.0229) -> (-198.3214, -4.1852) centre (-198.1245, -4.2199) ccw construction
  line L347 (-180.5601, -7.1135) -> (-198.0898, -4.0229) construction
  arc A163 (-180.3979, -7.3452) -> (-180.5601, -7.1135) centre (-180.5948, -7.3105) ccw construction
  line L348 (-183.4884, -24.8748) -> (-180.3979, -7.3452) construction
  line L349 (-199.3615, -20.4517) -> (-184.9833, -22.9866) construction
  line L350 (-184.9833, -22.9866) -> (-182.4483, -8.6084) construction
  line L351 (-182.4483, -8.6084) -> (-196.8266, -6.0734) construction
  line L352 (-196.8266, -6.0734) -> (-199.3615, -20.4517) construction
  arc A164 (-55.2481, -44.669) -> (-55.0164, -44.8312) centre (-55.0512, -44.6342) ccw construction
  line L353 (-58.339, -27.1394) -> (-55.2481, -44.669) construction
  arc A165 (-58.1767, -26.9077) -> (-58.339, -27.1394) centre (-58.142, -27.1046) ccw construction
  line L354 (-40.6471, -23.8168) -> (-58.1767, -26.9077) construction
  arc A166 (-40.4154, -23.9791) -> (-40.6471, -23.8168) centre (-40.6124, -24.0138) ccw construction
  line L355 (-41.9103, -25.8673) -> (-56.2885, -28.4025) construction
  line L356 (-56.2885, -28.4025) -> (-53.7533, -42.7807) construction
  arc A167 (-45.9204, 11.7993) -> (-45.6888, 11.6371) centre (-45.7235, 11.834) ccw construction
  line L357 (-49.0113, 29.3289) -> (-45.9204, 11.7993) construction
  arc A168 (-48.849, 29.5606) -> (-49.0113, 29.3289) centre (-48.8143, 29.3636) ccw construction
  line L358 (-46.9608, 28.0657) -> (-44.4256, 13.6875) construction
  line L359 (-189.2012, 53.3044) -> (-151.778, 46.7065)
  line L360 (-151.778, 46.7065) -> (-151.2572, 49.6608)
  line L361 (-151.2572, 49.6608) -> (-132.5457, 46.3619)
  line L362 (-132.5457, 46.3619) -> (-131.6776, 51.2859)
  line L363 (-131.6776, 51.2859) -> (-111.7844, 47.7786)
  line L364 (-111.7844, 47.7786) -> (-112.8262, 41.8696)
  line L365 (-112.8262, 41.8696) -> (-94.1148, 38.5707)
  line L366 (-94.1148, 38.5707) -> (-94.983, 33.6466)
  line L367 (-94.983, 33.6466) -> (-76.2716, 30.3477)
  line L368 (-76.2716, 30.3477) -> (-82.3476, -4.1158)
  line L369 (-82.3476, -4.1158) -> (-63.6397, -7.4141)
  line L370 (-189.2012, 53.3044) -> (-202.6052, -22.723)
  line L371 (-202.6052, -22.723) -> (-164.0005, -29.5291)
  line L372 (-164.0005, -29.5291) -> (-163.4797, -26.5749)
  line L373 (-163.4797, -26.5749) -> (-144.826, -29.8637)
  line L374 (-144.826, -29.8637) -> (-143.9578, -24.9397)
  line L375 (-143.9578, -24.9397) -> (-126.3705, -28.0404)
  line L376 (-126.3705, -28.0404) -> (-127.4123, -33.9494)
  line L377 (-127.4123, -33.9494) -> (-108.7009, -37.2483)
  line L378 (-108.7009, -37.2483) -> (-109.5691, -42.1725)
  line L379 (-109.5691, -42.1725) -> (-89.6759, -45.6797)
  line L380 (-89.1521, -42.709) -> (-70.4439, -46.0074)
  line L381 (-89.6759, -45.6797) -> (-89.1521, -42.709)
  line L382 (-63.6397, -7.4141) -> (-70.4439, -46.0074)
  point P0 (0, 0)
  point P1 (-31.7507, 36.1092)
  point P2 (19.3285, -28.6462)
  point P3 (-17.1634, -39.7096)
  point P4 (-126.299, -0.001)
  point P5 (-94.5489, 36.1086)
  point P6 (-145.627, -28.6475)
  point P7 (-109.135, -39.7104)
  dimension "d8" = 1
  dimension "d9" = 1
  dimension "d10" = 1
  dimension "d11" = 1
  dimension "d12" = 1
  dimension "d13" = 1
  dimension "d14" = 1
  dimension "d15" = 1
  dimension "d16" = 1
  dimension "d17" = 1
  dimension "d18" = 1
  dimension "d19" = 1
  dimension "d20" = 1
  dimension "d21" = 1
  dimension "d22" = 1
  dimension "d23" = 1
  dimension "d24" = 1
  dimension "d25" = 1
  dimension "d26" = 1
  dimension "d27" = 1
  dimension "d28" = 1
  dimension "d32" = 1
  dimension "d33" = 1
  dimension "d34" = 1
  constraints: 334 end point, 272 symmetric about line, 123 point on circle, 61 centre point, 24 parallel, 10 perpendicular, 2 midpoint, 64 other
  measures "d8" distance between parallel lines of L10 L216
  measures "d9" distance between parallel lines of L17 L217
  measures "d10" distance between parallel lines of L18 L218
  measures "d11" distance between parallel lines of L25 L219
  measures "d12" distance between parallel lines of L26 L220
  measures "d13" distance between parallel lines of L27 L221
  measures "d14" distance between parallel lines of L34 L222
  measures "d15" distance from line of point (-31.751, 36.109) L35
  measures "d16" distance between parallel lines of L42 L224
  measures "d17" distance between parallel lines of L43 L225
  measures "d18" distance between parallel lines of L226 L58
  measures "d19" distance between parallel lines of L105 L227
  measures "d20" distance between parallel lines of L104 L228
  measures "d21" distance from line of L99 L228.end
  measures "d22" distance between parallel lines of L88 L230
  measures "d23" distance from line of L231 point (19.328, -28.646)
  measures "d24" distance between parallel lines of L80 L232
  measures "d25" distance between parallel lines of L73 L233
  measures "d26" distance between parallel lines of L72 L234
  measures "d27" distance from line of L65 point (-17.163, -39.71)
  measures "d28" distance between parallel lines of L64 L236
  measures "d32" distance between parallel lines of L67 L238
  measures "d33" distance between parallel lines of L48 L237
  measures "d34" distance between parallel lines of L59 L239
extrude "Extrusion2" cut sketch "Sketch2" against normal through all
sketch "Sketch4" plane through (0, 0, 0) normal (0, 0, -1) x (-1, 0, 0)
  line L0 (84.9894, -32.0688) -> (-24.7678, -55.0813) projected
  line L1 (-24.7678, -55.0813) -> (-101.5302, -55.0813) projected
  line L2 (-101.5302, -55.0813) -> (-211.2876, -32.0693) projected
  line L3 (-214.4061, -27.4599) -> (-199.0739, 59.5042) projected
  line L4 (-195.1347, 62.8097) -> (68.8351, 62.8097) projected
  line L5 (72.7744, 59.5042) -> (88.1078, -27.4594) projected
  line L6 (-6.411, -43.0585) -> (-5.3851, -47.9513) projected
  line L7 (-4.2011, -48.7248) -> (58.4367, -35.5909) projected
  line L8 (59.2102, -34.407) -> (58.1845, -29.515) projected
  line L9 (58.1845, -29.515) -> (78.609, -25.2326) projected
  line L10 (79.3886, -24.0803) -> (65.6244, 53.9833) projected
  line L11 (64.6396, 54.8097) -> (45.1392, 54.8097) projected
  line L12 (45.1392, 54.8097) -> (45.1392, 59.8097) projected
  line L13 (44.1392, 60.8097) -> (-19.8608, 60.8097) projected
  line L14 (-20.8608, 59.8097) -> (-20.8608, 54.8097) projected
  line L15 (-20.8608, 54.8097) -> (-105.4391, 54.8097) projected
  line L16 (-105.4391, 54.8097) -> (-105.4391, 59.8097) projected
  line L17 (-106.4391, 60.8097) -> (-170.4391, 60.8097) projected
  line L18 (-171.4391, 59.8097) -> (-171.4391, 54.8097) projected
  line L19 (-171.4391, 54.8097) -> (-190.9391, 54.8097) projected
  line L20 (-191.9239, 53.9833) -> (-205.6869, -24.0807) projected
  line L21 (-204.9073, -25.2331) -> (-184.4826, -29.5154) projected
  line L22 (-184.4826, -29.5154) -> (-185.5086, -34.409) projected
  line L23 (-184.7351, -35.5929) -> (-122.097, -48.7257) projected
  line L24 (-120.9131, -47.9522) -> (-119.8871, -43.0586) projected
  line L25 (-119.8871, -43.0586) -> (-100.7006, -47.0813) projected
  line L26 (-100.7006, -47.0813) -> (-25.5975, -47.0813) projected
  line L27 (-25.5975, -47.0813) -> (-6.411, -43.0585) projected
  arc A0 (84.9894, -32.0688) -> (88.1078, -27.4594) centre (84.1686, -28.1539) ccw projected
  arc A1 (-214.4061, -27.4599) -> (-211.2876, -32.0693) centre (-210.4668, -28.1544) ccw projected
  arc A2 (-195.1347, 62.8097) -> (-199.0739, 59.5042) centre (-195.1347, 58.8097) ccw projected
  arc A3 (72.7744, 59.5042) -> (68.8351, 62.8097) centre (68.8351, 58.8097) ccw projected
  arc A4 (-5.3851, -47.9513) -> (-4.2011, -48.7248) centre (-4.4064, -47.7461) ccw projected
  arc A5 (58.4367, -35.5909) -> (59.2102, -34.407) centre (58.2315, -34.6122) ccw projected
  arc A6 (78.609, -25.2326) -> (79.3886, -24.0803) centre (78.4038, -24.2539) ccw projected
  arc A7 (65.6244, 53.9833) -> (64.6396, 54.8097) centre (64.6396, 53.8097) ccw projected
  arc A8 (45.1392, 59.8097) -> (44.1392, 60.8097) centre (44.1392, 59.8097) ccw projected
  arc A9 (-19.8608, 60.8097) -> (-20.8608, 59.8097) centre (-19.8608, 59.8097) ccw projected
  arc A10 (-105.4391, 59.8097) -> (-106.4391, 60.8097) centre (-106.4391, 59.8097) ccw projected
  arc A11 (-170.4391, 60.8097) -> (-171.4391, 59.8097) centre (-170.4391, 59.8097) ccw projected
  arc A12 (-190.9391, 54.8097) -> (-191.9239, 53.9833) centre (-190.9391, 53.8097) ccw projected
  arc A13 (-205.6869, -24.0807) -> (-204.9073, -25.2331) centre (-204.7021, -24.2544) ccw projected
  arc A14 (-185.5086, -34.409) -> (-184.7351, -35.5929) centre (-184.5299, -34.6142) ccw projected
  arc A15 (-122.097, -48.7257) -> (-120.9131, -47.9522) centre (-121.8918, -47.747) ccw projected
extrude "Extrusion4" cut sketch "Sketch4" against normal blind 2 contours L27 L26 L25 L24 A15 L23 A14 L22 L21 A13 L20 A12 L19 L18 A11 L17 A10 L16 L15 L14 A9 L13 A8 L12 L11 A7 L10 A6 L9 L8 A5 L7 A4 L6
fillet "Fillet1" radius 4 4 edges at (-72.1915, 62.8097, 3.5) (-88.7804, -31.274, 3.5) (198.4911, 62.8097, 3.5) (215.0786, -31.2745, 3.5)